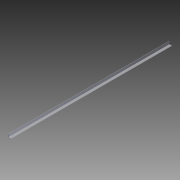
# Autodesk Inventor part: long angle rail
Saved by Autodesk Inventor 2012 (Build 160160000, 160)
## iProperties
Created: 2013-05-11
Part Number: long angle rail
Material: Default
Document SubType Name: Modeling
Designer: Fabian
Density: 1 g/cm^3
Author: Fabian
Autodesk Inventor part; units mm, degrees
ref_plane "YZ Plane" through (0, 0, 0) normal (1, 0, 0) x (0, 1, 0)
ref_plane "XZ Plane" through (0, 0, 0) normal (0, 1, 0) x (-1, 0, 0)
ref_plane "XY Plane" through (0, 0, 0) normal (0, 0, 1) x (1, 0, 0)
sketch "Sketch1" plane through (0, 0, 0) normal (0, 0, 1) x (1, 0, 0)
  line L0 (-13.007, 33.4846) -> (-9.832, 33.4846)
  line L1 (-9.832, 33.4846) -> (-9.832, -4.6154)
  line L2 (-9.832, -4.6154) -> (-13.007, -4.6154)
  line L3 (-13.007, -4.6154) -> (-13.007, 33.4846)
  line L4 (-9.832, -4.6154) -> (25.093, -4.6154)
  line L5 (25.093, -4.6154) -> (25.093, -1.4404)
  line L6 (25.093, -1.4404) -> (-9.832, -1.4404)
  line L7 (-9.832, -1.4404) -> (-9.832, -4.6154)
  point P0 (0, 0)
  dimension "d2" = 38.1
  dimension "d3" = 38.1
  dimension "d4" = 3.175
  dimension "d5" = 3.175
  constraints: 16 end point, 4 parallel, 2 horizontal, 2 perpendicular
  measures "d2" distance between parallel lines of L5 L3
  measures "d3" distance of L2.end L0.start
  measures "d4" distance between parallel lines of L1 L3
  measures "d5" distance between parallel lines of L6 L4
extrude "Extrusion1" add sketch "Sketch1" along normal blind 2133.6
body "Solid1"
